post_mount (Autodesk Fusion 360 design; units mm, degrees)
Autodesk Fusion 360 part; units mm, degrees
note: some values were not read from the file. Chosen so that the rebuilt part matches the saved one: that a step has no effect.
sketch "Sketch1" plane through (0, 0, 0) normal (0, 0, 1) x (1, 0, 0)
  line L0 (0, 0) -> (9.2, 0)
  line L1 (9.2, 0) -> (9.2, 9.2)
  line L2 (9.2, 9.2) -> (0, 9.2)
  line L3 (0, 9.2) -> (0, 0)
  line L4 (-3, 12.2) -> (12, 12.2)
  line L5 (12, 12.2) -> (12, -2.8)
  line L6 (12, -2.8) -> (-3, -2.8)
  line L7 (-3, -2.8) -> (-3, 12.2)
  line L8 (-3, -17.8) -> (12, -17.8)
  line L9 (12, -17.8) -> (12, 27.2)
  line L10 (12, 27.2) -> (-3, 27.2)
  line L11 (-3, 27.2) -> (-3, -17.8)
  line L12 (-18, 12.2) -> (27, 12.2)
  line L13 (27, 12.2) -> (27, -2.8)
  line L14 (27, -2.8) -> (-18, -2.8)
  line L15 (-18, -2.8) -> (-18, 12.2)
  line L16 (-18, 4.7) -> (27, 4.7) construction
  line L17 (4.5, 27.2) -> (4.5, -17.8) construction
  circle A0 centre (-13, 4.7) radius 1.7
  circle A1 centre (4.5, 22.2) radius 1.7
  circle A2 centre (22, 4.7) radius 1.7
  circle A3 centre (4.5, -12.8) radius 1.7
  line L18 (9.2, 0) -> (15.2, 0)
  line L19 (15.2, 0) -> (15.2, 10.3)
  line L20 (15.2, 10.3) -> (9.2, 10.3)
  line L21 (9.2, 10.3) -> (9.2, 0)
  line L22 (18.2, 12.2) -> (18.2, -2.8)
  line L23 (15.2, 0) -> (14.2, 0)
  line L24 (14.2, 0) -> (14.2, 10.3)
  line L25 (14.2, 10.3) -> (15.2, 10.3)
  line L26 (15.2, 10.3) -> (15.2, 0)
  line L27 (9.2, 0) -> (10.2, 0)
  line L28 (10.2, 0) -> (10.2, 10.3)
  line L29 (10.2, 10.3) -> (9.2, 10.3)
  line L30 (9.2, 10.3) -> (9.2, 0)
  dimension "d1" = 9.2
  dimension "d2" = 9.2
  dimension "d3" = 15
  dimension "d4" = 15
  dimension "d5" = 3
  dimension "d6" = 3
  dimension "d7" = 15
  dimension "d8" = 15
  dimension "d9" = 15
  dimension "d10" = 15
  dimension "d11" = 3.4
  dimension "d12" = 10
  dimension "d13" = 3.4
  dimension "d14" = 3.4
  dimension "d15" = 3.4
  dimension "d16" = 10
  dimension "d17" = 10
  dimension "d18" = 10
  dimension "d33" = 6
  dimension "d34" = 10.3
  dimension "d44" = 3
  dimension "d71" = 1
  dimension "d72" = 10.3
  dimension "d73" = 1
  dimension "d74" = 10.3
  constraint horizontal L0
  constraint vertical L1
  constraint horizontal L2
  constraint vertical L3
  constraint coincident L0.start L3.end
  constraint horizontal L4
  constraint vertical L5
  constraint horizontal L6
  constraint vertical L7
  constraint horizontal L8
  constraint vertical L9
  constraint horizontal L10
  constraint vertical L11
  constraint horizontal L12
  constraint vertical L13
  constraint horizontal L14
  constraint vertical L15
  constraint midpoint L15 L16.start
  constraint midpoint L13 L16.end
  constraint midpoint L10 L17.start
  constraint midpoint L8 L17.end
  constraint coincident L16 A0.centre
  constraint coincident L17 A1.centre
  constraint coincident L16 A2.centre
  constraint coincident L17 A3.centre
  constraint coincident L4.end L12
  constraint coincident L5.end L14
  constraint coincident L4.end L9
  constraint coincident L4.start L11
  constraint horizontal L18
  constraint vertical L19
  constraint horizontal L20
  constraint vertical L21
  constraint coincident L12 L22.start
  constraint coincident L14 L22.end
  constraint perpendicular L14 L22
  constraint horizontal L23
  constraint vertical L24
  constraint horizontal L25
  constraint vertical L26
  constraint horizontal L27
  constraint vertical L28
  constraint horizontal L29
  constraint vertical L30
  measures "d1" distance of L0.start L0.end
  measures "d2" distance of L0.start L2.end
  measures "d3" distance of L4.start L4.end
  measures "d4" distance of L4.start L6.end
  measures "d5" distance of L3 L7
  measures "d6" distance of L2 L4
  measures "d7" distance of L5.end L13.end
  measures "d8" distance of L6.end L14.end
  measures "d9" distance of L4.end L9.end
  measures "d10" distance of L5.end L8.end
  measures "d11" diameter of A0
  measures "d12" distance of L7 A0.centre
  measures "d13" diameter of A1
  measures "d14" diameter of A2
  measures "d15" diameter of A3
  measures "d16" distance of L12 A1.centre
  measures "d17" distance of L9 A2.centre
  measures "d18" distance of L14 A3.centre
  measures "d33" distance of L0.end L18.end
  measures "d34" distance of L0.end L20.end
  measures "d44" distance of L19 L22
  measures "d71" distance of L18.end L23.end
  measures "d72" distance of L18.end L19.end
  measures "d73" distance of L0.end L27.end
  measures "d74" distance of L0.end L20.end
extrude "Extrude1" add sketch "Sketch1" along normal blind 2 contours L0 L2 L3 L4 L5 L6 L7 L9 L11 L12 L14 L18 L20 L21 L27 L29 L30 | L1 L18 L20 L21 L27 L28 L29 L30 | L5 L9 L18 L20 L28 makes body 1
extrude "Extrude4" add sketch "Sketch1" along normal blind 3 separate body contours L5 L9 L12 L14 L18 L19 L20 L22 L23 L25 L26 | L4 L9 L10 L11 L12 | L7 L11 L12 L14 L15 | L12 L13 L14 L22 makes body 2 at (21.3577, 9.6317, 0)
extrude "Extrude5" add sketch "Sketch1" along normal blind 3 contours L6 L8 L9 L11 L14 bodies 1 2
extrude "Extrude6" cut sketch "Sketch1" along normal through all contours L1 L18 L20 L21 L27 L28 L29 L30 | L5 L9 L18 L20 L28 bodies 1
extrude "Extrude7" add 1 faces at (-2, 6.2, 2) along direction (0, 0, 1) blind 5 on bodies 1 bodies 1
extrude "Extrude8" add 1 faces at (-2, 6.2, 7) along direction (0, 0, 1) blind 1 on bodies 1 bodies 1
copy_body "CopyPasteBodies1" bodies 1 makes body 3
extrude "Extrude9" add sketch "Sketch1" along normal blind 3 contours L5 L9 L18 L20 L24 | L18 L19 L20 L23 L24 L25 L26 bodies 1 3
extrude "Extrude10" add sketch "Sketch1" along normal blind 8 contours L1 L18 L20 L21 L27 L28 L29 L30 | L5 L9 L18 L20 L28 bodies 1
sketch "Sketch6" plane through (0, 0, 3) normal (0, 0, 1) x (-1, 0, 0)
  circle A0 centre (-22, -4.7) radius 1.7
  line L0 (-12, -12.2) -> (-12, 2.8)
  line L1 (-12, 2.8) -> (-27, 2.8)
  line L2 (-27, 2.8) -> (-27, -12.2)
  line L3 (-27, -12.2) -> (-12, -12.2)
  circle A1 centre (-4.5, 12.8) radius 1.7
  line L4 (-12, 17.8) -> (-12, 2.8)
  line L5 (-12, 2.8) -> (3, 2.8)
  line L6 (3, 2.8) -> (3, 17.8)
  line L7 (3, 17.8) -> (-12, 17.8)
  circle A2 centre (13, -4.7) radius 1.7
  line L8 (18, 2.8) -> (3, 2.8)
  line L9 (3, 2.8) -> (3, -12.2)
  line L10 (3, -12.2) -> (18, -12.2)
  line L11 (18, -12.2) -> (18, 2.8)
  circle A3 centre (-4.5, -22.2) radius 1.7
  line L12 (3, -27.2) -> (3, -12.2)
  line L13 (3, -12.2) -> (-12, -12.2)
  line L14 (-12, -12.2) -> (-12, -27.2)
  line L15 (-12, -27.2) -> (3, -27.2)
hole "Hole2" at (4.5, -12.8, 3) at (22, 4.7, 3) at (4.5, 22.2, 3) at (-13, 4.7, 3) direction (0, 0, -1) diameter 3.4 depth 6 tip angle 180 countersink diameter 6.3 countersink angle 90 bodies 1
fillet "Fillet1" radius 3 1 edges at (4.5, 12.2, 3) on bodies 1
fillet "Fillet2" [no effect]
fillet "Fillet3" [no effect]
fillet "Fillet4" radius 3 1 edges at (12, 4.7, 3) on bodies 1
copy_body "CopyPasteBodies2" bodies 1 makes body 4
move_body "Move1" bodies 4 to x (1, 0, 0) y (0, 1, 0) z (0, 0, 1) at (55, 0, 0)
extrude "Extrude11" cut sketch "Sketch1" along normal through all contours L1 L18 L20 L21 L27 L28 L29 L30 | L5 L9 L18 L20 L28 | L5 L9 L18 L20 L24 | L18 L19 L20 L23 L24 L25 L26 bodies 1
extrude "Extrude12" add sketch "Sketch1" along normal blind 8 contours L5 L9 L12 L14 L18 L19 L20 L22 L23 L25 L26 bodies 1
extrude "Extrude13" add sketch "Sketch1" along normal blind 1 contours L0 L1 L2 L3 L21 L30 | L1 L18 L20 L21 L27 L28 L29 L30 | L5 L9 L18 L20 L28 | L5 L9 L18 L20 L24 | L18 L19 L20 L23 L24 L25 L26 bodies 1
sketch "Sketch7" plane through (0, 0, 0) normal (0, 0, -1) x (1, 0, 0)
  line L0 (67, -12.2) -> (82, -12.2)
  line L1 (82, -12.2) -> (82, 2.8)
  line L2 (82, 2.8) -> (67, 2.8)
  line L3 (67, 2.8) -> (67, 17.8)
  line L4 (67, 17.8) -> (52, 17.8)
  line L5 (52, 17.8) -> (52, 2.8)
  line L6 (37, 2.8) -> (37, -12.2)
  line L7 (37, -12.2) -> (52, -12.2)
  line L8 (52, -12.2) -> (52, -27.2)
  line L9 (52, -27.2) -> (67, -27.2)
  line L10 (67, -27.2) -> (67, -12.2)
  circle A0 centre (77, -4.7) radius 1.7
  line L11 (55, 0) -> (64.2, 0)
  line L12 (64.2, 0) -> (64.2, -9.2)
  line L13 (64.2, -9.2) -> (55, -9.2)
  line L14 (55, -9.2) -> (55, 0)
  circle A1 centre (59.5, -22.2) radius 1.7
  circle A2 centre (42, -4.7) radius 1.7
  circle A3 centre (59.5, 12.8) radius 1.7
  line L15 (64.2, -9.2) -> (55, -9.2)
  line L16 (55, -9.2) -> (55, 0)
  line L17 (55, 0) -> (64.2, 0)
  line L18 (64.2, 0) -> (64.2, -9.2)
  line L19 (52, 2.8) -> (37, 2.8)
  constraint horizontal L15
  constraint vertical L16
  constraint horizontal L17
  constraint vertical L18
  constraint coincident L11.start L14.end
  constraint coincident L12.end L13.start
extrude "Extrude14" add sketch "Sketch7" against normal blind 1 contours L11 L12 L13 L14 L15 L16 L17 L18 bodies 4
extrude "Extrude15" cut sketch "Sketch1" along normal blind 1 contours L1 L18 L20 L21 L27 L28 L29 L30 | L5 L9 L18 L20 L28 | L5 L9 L18 L20 L24 | L18 L19 L20 L23 L24 L25 L26 bodies 1
sketch "Sketch8" plane through (9.2, 0, 0) normal (1, 0, 0) x (0, 1, 0)
  line L0 (10.3, 0) -> (10.3, 8)
  line L1 (10.3, 8) -> (9.2, 8)
  line L2 (9.2, 8) -> (9.2, 1)
  line L3 (9.2, 1) -> (0, 1)
  line L4 (0, 1) -> (0, 0)
  line L5 (0, 0) -> (10.3, 0)
extrude "Extrude16" add sketch "Sketch1" along normal blind 1 contours L1 L18 L20 L21 L27 L28 L29 L30 | L18 L19 L20 L23 L24 L25 L26 bodies 1
fillet "Fillet5" radius 3 1 edges at (-3, 4.7, 3) on bodies 1
fillet "Fillet6" radius 3 1 edges at (4.5, -2.8, 3) on bodies 1
fillet "Fillet7" radius 3 1 edges at (59.5, -2.8, 3) on bodies 4
fillet "Fillet8" radius 3 1 edges at (52, 4.7, 3) on bodies 4
